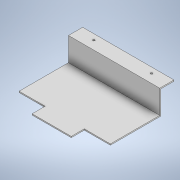
# Autodesk Inventor part: Plate
Saved by Autodesk Inventor 2020 (Build 240168000, 168)
## iProperties
Created: 2020-12-02
Part Number: Plate
Material: Generic
Document SubType Name: Modeling
Designer: tdmp4
Density: 1 g/cm^3
Appearance: Default
Author: tdmp4
Autodesk Inventor part; units mm, degrees
ref_plane "YZ Plane" through (0, 0, 0) normal (1, 0, 0) x (0, 1, 0)
ref_plane "XZ Plane" through (0, 0, 0) normal (0, 1, 0) x (-1, 0, 0)
ref_plane "XY Plane" through (0, 0, 0) normal (0, 0, 1) x (1, 0, 0)
sketch "Sketch1" plane through (0, 0, 0) normal (1, 0, 0) x (0, 1, 0)
  line L0 (0, 0) -> (2.286, 0)
  line L1 (2.286, 0) -> (2.286, -25.4)
  line L2 (2.286, -25.4) -> (0, -25.4)
  line L3 (0, -25.4) -> (0, 0)
  line L4 (0, 0) -> (-45.974, 0)
  line L5 (-45.974, 0) -> (-45.974, 123.825)
  line L6 (-45.974, 123.825) -> (-43.688, 123.825)
  line L7 (-43.688, 123.825) -> (-43.688, 0)
  line L8 (-45.974, 0) -> (-45.974, 2.286)
  line L9 (-45.974, 2.286) -> (2.286, 2.286)
  line L10 (2.286, 2.286) -> (2.286, 0)
  point P0 (-43.688, 2.286)
  dimension "d0" = 25.4
  dimension "d1" = 2.286
  dimension "d4" = 2.286
  dimension "d5" = 2.286
  constraints: 22 end point, 5 perpendicular, 3 horizontal, 2 parallel, 2 point on line
  measures "d0" distance of L0.end L1.end
  measures "d1" distance of L1.end L2.end
  measures "d4" distance of L5.end L6.end
  measures "d5" distance of L4.end L8.end
extrude "Extrusion1" add sketch "Sketch1" along normal blind 177.8
sketch "Sketch2" plane through (0, -43.688, 123.825) normal (0, 1, 0) x (1, 0, 0)
  line L0 (0, 0) -> (177.8, 0) projected
  line L1 (0, 0) -> (50.8, 0)
  line L2 (50.8, 0) -> (50.8, 25.4)
  line L3 (50.8, 25.4) -> (0, 25.4)
  line L4 (0, 25.4) -> (0, 0)
  line L5 (177.8, 0) -> (127, 0)
  line L6 (127, 0) -> (127, 25.4)
  line L7 (127, 25.4) -> (177.8, 25.4)
  line L8 (177.8, 25.4) -> (177.8, 0)
  point P0 (0, 123.825)
  point P1 (50.8, 0)
  point P2 (127, 0)
  dimension "d8" = 50.8
  dimension "d9" = 25.4
  dimension "d10" = 50.8
  constraints: 16 end point, 4 parallel, 2 horizontal, 2 perpendicular
  measures "d8" distance of L2.end L3.end
  measures "d9" distance of L1.end L2.end
  measures "d10" distance of L6.end L7.end
extrude "Extrusion2" cut sketch "Sketch2" against normal blind 177.8
sketch "Sketch4" plane through (0, 2.286, 2.286) normal (0, 1, 0) x (1, 0, 0)
  line L0 (0, 2.286) -> (0, 27.686) projected
  line L1 (0, 16.6049) -> (177.8, 16.7157)
  line L2 (177.8, 27.686) -> (177.8, 0) projected
  circle A0 centre (32.7282, 16.6253) radius 1.905
  line L3 (0, 27.686) -> (177.8, 27.686) projected
  line L4 (0, 0) -> (177.8, 0) projected
  line L5 (177.8, 27.686) -> (145.0594, 27.686)
  line L6 (145.0594, 27.686) -> (145.0594, 0)
  line L7 (145.0594, 0) -> (177.8, 0)
  line L8 (177.8, 0) -> (177.8, 27.686)
  circle A1 centre (145.0594, 16.6953) radius 1.905
  dimension "d13" = 3.81
  dimension "d14" = 32.7406
  dimension "d15" = 3.81
  constraints: 10 end point, 6 point on line, 2 centre point, 2 parallel, 1 horizontal, 1 perpendicular
  measures "d13" diameter of A0
  measures "d14" distance of L7.end L6.end
  measures "d15" diameter of A1
extrude "Extrusion3" cut sketch "Sketch4" against normal blind 177.8 contours A0 L1 | L1 A0 | A1 L1 L6 | L6 L1 A1 | L1 L6 A1 | L1 A1 L6
body "Solid1"
